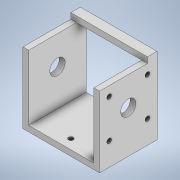
# Autodesk Inventor part: 3SR02_振子支え
Saved by Autodesk Inventor 2021 (Build 250183000, 183)
## iProperties
Created: 2021-04-19
Part Number: 3SR02_振子支え
Material: 一般
Document SubType Name: Modeling
Designer: ryusei
Density: 1 g/cm^3
Appearance: 既定
Author: ryusei
Autodesk Inventor part; units mm, degrees
ref_plane "YZ Plane" through (0, 0, 0) normal (1, 0, 0) x (0, 1, 0)
ref_plane "XZ Plane" through (0, 0, 0) normal (0, 1, 0) x (-1, 0, 0)
ref_plane "XY Plane" through (0, 0, 0) normal (0, 0, 1) x (1, 0, 0)
sketch "スケッチ1" plane through (0, 0, 0) normal (0, 0, 1) x (1, 0, 0)
  line L0 (0, 0) -> (40, 0)
  line L1 (40, 0) -> (40, 40)
  line L2 (40, 40) -> (0, 40)
  line L3 (0, 40) -> (0, 0)
  dimension "d0" = 40
  dimension "d1" = 40
  constraints: 8 end point, 2 parallel, 1 horizontal, 1 perpendicular
  measures "d0" distance between parallel lines of L1 L3
  measures "d1" distance between parallel lines of L0 L2
extrude "押し出し1" add sketch "スケッチ1" along normal blind 40
sketch "スケッチ2" plane through (0, 0, 0) normal (0, 0, -1) x (-1, 0, 0)
  point P0 (0, 0)
sketch "スケッチ3" plane through (0, 0, 40) normal (0, 0, 1) x (1, 0, 0)
  line L0 (3, 3) -> (37, 3)
  line L1 (37, 3) -> (37, 37)
  line L2 (37, 37) -> (3, 37)
  line L3 (3, 37) -> (3, 3)
  line L4 (0, 40) -> (0, 0) projected
  line L5 (40, 40) -> (0, 40) projected
  line L6 (40, 0) -> (40, 40) projected
  line L7 (0, 0) -> (40, 0) projected
  dimension "d4" = 3
  dimension "d5" = 3
  dimension "d6" = 3
  dimension "d7" = 3
  constraints: 8 end point, 2 parallel, 1 horizontal, 1 perpendicular
  measures "d4" distance between parallel lines of L3 L4
  measures "d5" distance between parallel lines of L5 L2
  measures "d6" distance between parallel lines of L6 L1
  measures "d7" distance between parallel lines of L7 L0
extrude "押し出し2" cut sketch "スケッチ3" against normal through all contours L3 L2 L1 L0
sketch "スケッチ4" plane through (0, 40, 0) normal (0, 1, 0) x (1, 0, 0)
  line L0 (0, 0) -> (0, -40) projected
  line L1 (40, 0) -> (40, -40) projected
  line L2 (0, -40) -> (40, -40)
  line L3 (40, -40) -> (40, -5)
  line L4 (40, -5) -> (0, -5)
  line L5 (0, -5) -> (0, -40)
  line L6 (40, 0) -> (0, 0) projected
  point P0 (0, -5)
  dimension "d10" = 5
  constraints: 8 end point, 2 parallel, 1 horizontal, 1 perpendicular, 1 point on line
  measures "d10" distance between parallel lines of L6 L4
extrude "押し出し3" cut sketch "スケッチ4" against normal blind 3 contours L4 L1 L2 L0
sketch "スケッチ5" plane through (0, 0, 0) normal (0, -1, 0) x (1, 0, 0)
  line L0 (0, 40) -> (0, 5) projected
  line L1 (0, 30) -> (40, 30)
  line L2 (40, 5) -> (40, 40) projected
  line L3 (0, 40) -> (40, 40) projected
  point P0 (0, 0)
  dimension "d13" = 10
  constraints: 2 end point, 2 point on line, 1 horizontal
  measures "d13" distance between parallel lines of L1 L3
extrude "押し出し4" cut sketch "スケッチ5" against normal through all
sketch "スケッチ6" plane through (0, 37, 0) normal (0, 1, 0) x (1, 0, 0)
  point P0 (0, 0)
sketch "スケッチ7" plane through (0, 0, 0) normal (0, -1, 0) x (1, 0, 0)
  line L0 (40, 30) -> (0, 30) projected
  line L1 (0, 0) -> (40, 0) projected
  line L2 (40, 0) -> (40, 30) projected
  point P0 (20, 5)
  point P1 (20, 25)
  dimension "d16" = 5
  dimension "d17" = 5
  dimension "d18" = 20
  dimension "d19" = 20
  measures "d16" distance from line of L1 point (20, 5)
  measures "d17" distance from line of L0 point (20, 25)
  measures "d18" distance from line of L2 point (20, 25)
  measures "d19" distance from line of L2 point (20, 5)
hole "穴1" at (20, 0, 5) at (20, 0, 25) direction (0, 1, 0) diameter 2.459 depth 3 thread size "M3x0.5" class "6H" standard "ANSI Metric M Profile"
sketch "スケッチ8" plane through (40, 0, 0) normal (1, 0, 0) x (0, 0, -1)
  line L0 (-30, 37) -> (-30, 0) projected
  line L1 (-5, 37) -> (-30, 37) projected
  line L2 (0, 0) -> (-30, 0) projected
  line L3 (0, 0) -> (0, 40) projected
  line L4 (0, 40) -> (-5, 40) projected
  point P0 (-25, 32)
  point P1 (-5, 32)
  point P2 (-5, 12)
  point P3 (-25, 12)
  dimension "d27" = 5
  dimension "d28" = 5
  dimension "d29" = 5
  dimension "d30" = 12
  dimension "d31" = 12
  dimension "d32" = 5
  dimension "d33" = 5
  dimension "d34" = 8
  measures "d27" distance from line of point (-25, 32) L0
  measures "d28" distance from line of L1 point (-25, 32)
  measures "d29" distance from line of L0 point (-25, 12)
  measures "d30" distance from line of L2 point (-25, 12)
  measures "d31" distance from line of L2 point (-5, 12)
  measures "d32" distance from line of L3 point (-5, 12)
  measures "d33" distance from line of L3 point (-5, 32)
  measures "d34" distance from line of L4 point (-5, 32)
hole "穴2" at (40, 32, 25) at (40, 32, 5) at (40, 12, 25) at (40, 12, 5) direction (-1, 0, 0) diameter 2.459 depth 3 thread size "M3x0.5" class "6H" standard "ANSI Metric M Profile"
sketch "スケッチ9" plane through (40, 0, 0) normal (1, 0, 0) x (0, 0, -1)
  line L0 (-30, 37) -> (-30, 0) projected
  line L1 (-5, 37) -> (-30, 37) projected
  line L2 (0, 0) -> (-30, 0) projected
  point P0 (-15, 22)
  dimension "d42" = 15
  dimension "d44" = 22
  measures "d42" distance from line of point (-15, 22) L0
  measures "d44" distance from line of point (-15, 22) L2
hole "穴3" at (40, 22, 15) direction (-1, 0, 0) diameter 8 end through all
